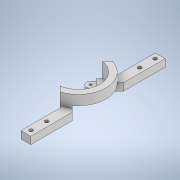
# Autodesk Inventor part: snHeadbarHolder2
Saved by Autodesk Inventor 2022 (Build 260153000, 153)
## iProperties
Created: 2022-02-24
Part Number: snHeadbarHolder2
Material: Generic
Document SubType Name: Modeling
Designer: misaa
Density: 1 g/cm^3
Appearance: Default
Author: misaa
Autodesk Inventor part; units mm, degrees
ref_plane "YZ Plane" through (0, 0, 0) normal (1, 0, 0) x (0, 1, 0)
ref_plane "XZ Plane" through (0, 0, 0) normal (0, 1, 0) x (-1, 0, 0)
ref_plane "XY Plane" through (0, 0, 0) normal (0, 0, 1) x (1, 0, 0)
sketch "Sketch1" plane through (0, 0, 0) normal (0, 1, 0) x (-1, 0, 0)
  arc A0 (-2.4004, 17.3346) -> (-2.3887, -17.3362) centre (0, 0) ccw
  arc A1 (-6.5816, 21.5159) -> (-6.5714, -21.519) centre (0, 0) ccw
  circle A2 centre (0, 10) radius 1
  circle A3 centre (0, -10) radius 1
  arc A4 (-2.3933, 7.4462) -> (2.2712, 12.663) centre (0, 10) ccw
  arc A5 (2.4002, -12.5474) -> (-2.4749, -7.5251) centre (0, -10) ccw
  line L0 (-8, 55) -> (-16, 55)
  line L1 (-16, -55) -> (-8, -55)
  line L2 (-8, -55) -> (-8, -22.9476)
  line L3 (-8, 22.9342) -> (-8, 55)
  line L4 (-16, -23.152) -> (-16, -55)
  line L5 (-8, 22.9342) -> (2.5474, 12.3868)
  line L6 (-8, 22.9342) -> (6.9163, 22.9342) construction
  line L7 (2.5474, -12.4002) -> (-8, -22.9476)
  line L8 (-2.4749, -7.5251) -> (-9.5993, -14.6496)
  circle A6 centre (-12, -50.8) radius 1.5
  circle A7 centre (-12, -38.1) radius 1.5
  circle A8 centre (-12, 50.8) radius 1.5
  circle A9 centre (-12, 38.1) radius 1.5
  line L9 (-16, 55) -> (-16, 21.0529)
  line L10 (-9.5993, -14.6496) -> (-16, -21.0503)
  line L11 (-16, -21.0503) -> (-16, -23.152)
  line L12 (-2.3933, 7.4462) -> (-16, 21.0529)
  line L13 (0, 14.9342) -> (-4.9407, 9.9935)
  line L14 (0, -14.9476) -> (-4.9487, -9.9989)
  point P0 (-9.5889, -14.6391)
  point P1 (-9.5873, 14.6401)
  dimension "d7" = 35
  dimension "d8" = 45
  dimension "d9" = 2
  dimension "d10" = 2
  dimension "d11" = 10
  dimension "d12" = 10
  dimension "d13" = 7
  dimension "d14" = 7
  dimension "d19" = 8
  dimension "d20" = 110
  dimension "d21" = 8
  dimension "d22" = 55
  dimension "d23" = 45
  dimension "d25" = 3
  dimension "d26" = 3
  dimension "d27" = 3
  dimension "d28" = 3
  dimension "d29" = 38.1
  dimension "d31" = 50.8
  constraints: 30 end point, 11 point on line, 10 centre point, 9 point on circle, 6 parallel, 4 coincident, 4 perpendicular, 2 horizontal, 1 equal length, 1 tangent, 1 vertical
  measures "d7" diameter of A0
  measures "d8" diameter of A1
  measures "d9" diameter of A2
  measures "d10" diameter of A3
  measures "d11" distance of point (0, 0) A2.centre
  measures "d12" distance of point (0, 0) A3.centre
  measures "d13" diameter of A4
  measures "d14" diameter of A5
  measures "d19" distance of L1.end L1.start
  measures "d20" distance of L1.start L0.end
  measures "d21" horizontal distance of point (0, 0) L1.end
  measures "d22" vertical distance of point (0, 0) L1.start
  measures "d23" angle of L5 L6
  measures "d25" diameter of A6
  measures "d26" diameter of A7
  measures "d27" diameter of A8
  measures "d28" diameter of A9
  measures "d29" vertical distance of point (0, 0) A7.centre
  measures "d31" vertical distance of A6.centre point (0, 0)
sketch "Sketch2" plane through (0, 0, 0) normal (0, 1, 0) x (-1, 0, 0)
  arc A0 (-2.4004, 17.3346) -> (-2.3887, -17.3362) centre (0, 0) ccw
  arc A1 (-6.5816, 21.5159) -> (-6.5714, -21.519) centre (0, 0) ccw
  circle A2 centre (0, 10) radius 1.13
  circle A3 centre (0, -10) radius 1.13
  arc A4 (-2.3933, 7.4462) -> (2.2712, 12.663) centre (0, 10) ccw
  arc A5 (2.4002, -12.5474) -> (-2.4749, -7.5251) centre (0, -10) ccw
  line L0 (-8, 55) -> (-16, 55)
  line L1 (-16, -55) -> (-8, -55)
  line L2 (-8, -55) -> (-8, -22.9476)
  line L3 (-8, 22.9342) -> (-8, 55)
  line L4 (-16, -23.152) -> (-16, -55)
  line L5 (-8, 22.9342) -> (2.5474, 12.3868)
  line L6 (-8, 22.9342) -> (6.9163, 22.9342) construction
  line L7 (2.5474, -12.4002) -> (-8, -22.9476)
  line L8 (-2.4749, -7.5251) -> (-9.5993, -14.6496)
  circle A6 centre (-12, -50.8) radius 1.5
  circle A7 centre (-12, -38.1) radius 1.5
  circle A8 centre (-12, 50.8) radius 1.5
  circle A9 centre (-12, 38.1) radius 1.5
  line L9 (-16, 55) -> (-16, 21.0529)
  line L10 (-9.5993, -14.6496) -> (-16, -21.0503)
  line L11 (-16, -21.0503) -> (-16, -23.152)
  line L12 (-2.3933, 7.4462) -> (-16, 21.0529)
  line L13 (0, 14.9342) -> (-4.9407, 9.9935)
  line L14 (0, -14.9476) -> (-4.9487, -9.9989)
  dimension "d54" = 35
  dimension "d55" = 45
  dimension "d56" = 2.26
  dimension "d57" = 2.26
  dimension "d58" = 10
  dimension "d59" = 10
  dimension "d60" = 7
  dimension "d61" = 7
  dimension "d62" = 8
  dimension "d63" = 110
  dimension "d64" = 8
  dimension "d65" = 55
  dimension "d66" = 45
  dimension "d67" = 3
  dimension "d68" = 3
  dimension "d69" = 3
  dimension "d70" = 3
  dimension "d71" = 38.1
  dimension "d72" = 50.8
  constraints: 30 end point, 11 point on line, 10 centre point, 9 point on circle, 6 parallel, 4 coincident, 4 perpendicular, 2 horizontal, 1 equal length, 1 tangent, 1 vertical
  measures "d54" diameter of A0
  measures "d55" diameter of A1
  measures "d56" diameter of A2
  measures "d57" diameter of A3
  measures "d58" distance of point (0, 0) A2.centre
  measures "d59" distance of point (0, 0) A3.centre
  measures "d60" diameter of A4
  measures "d61" diameter of A5
  measures "d62" distance of L1.end L1.start
  measures "d63" distance of L1.start L0.end
  measures "d64" horizontal distance of point (0, 0) L1.end
  measures "d65" vertical distance of point (0, 0) L1.start
  measures "d66" angle of L5 L6
  measures "d67" diameter of A6
  measures "d68" diameter of A7
  measures "d69" diameter of A8
  measures "d70" diameter of A9
  measures "d71" vertical distance of point (0, 0) A7.centre
  measures "d72" vertical distance of A6.centre point (0, 0)
sketch "Sketch3" plane through (0, 0, 0) normal (0, 1, 0) x (-1, 0, 0)
  arc A0 (-2.4004, 17.3346) -> (-2.3887, -17.3362) centre (0, 0) ccw
  arc A1 (-6.5816, 21.5159) -> (-6.5714, -21.519) centre (0, 0) ccw
  circle A2 centre (0, 10) radius 1
  circle A3 centre (0, -10) radius 1
  arc A4 (-2.3933, 7.4462) -> (2.2712, 12.663) centre (0, 10) ccw
  arc A5 (2.4002, -12.5474) -> (-2.4749, -7.5251) centre (0, -10) ccw
  line L0 (-8, 55) -> (-16, 55)
  line L1 (-16, -55) -> (-8, -55)
  line L2 (-8, -55) -> (-8, -22.9476)
  line L3 (-8, 22.9342) -> (-8, 55)
  line L4 (-16, -23.152) -> (-16, -55)
  line L5 (-8, 22.9342) -> (2.5474, 12.3868)
  line L6 (-8, 22.9342) -> (6.9163, 22.9342) construction
  line L7 (2.5474, -12.4002) -> (-8, -22.9476)
  line L8 (-2.4749, -7.5251) -> (-9.5993, -14.6496)
  circle A6 centre (-12, -50.8) radius 1.5
  circle A7 centre (-12, -38.1) radius 1.5
  circle A8 centre (-12, 50.8) radius 1.5
  circle A9 centre (-12, 38.1) radius 1.5
  line L9 (-16, 55) -> (-16, 21.0529)
  line L10 (-9.5993, -14.6496) -> (-16, -21.0503)
  line L11 (-16, -21.0503) -> (-16, -23.152)
  line L12 (-2.3933, 7.4462) -> (-16, 21.0529)
  line L13 (0, 14.9342) -> (-4.9407, 9.9935)
  line L14 (0, -14.9476) -> (-4.9487, -9.9989)
  point P0 (-9.5889, -14.6391)
  point P1 (-9.5873, 14.6401)
  point P2 (-13.1831, -18.2334)
  point P3 (-13.1816, 18.2345)
  dimension "d92" = 35
  dimension "d93" = 45
  dimension "d94" = 2
  dimension "d95" = 2
  dimension "d96" = 10
  dimension "d97" = 10
  dimension "d98" = 7
  dimension "d99" = 7
  dimension "d100" = 8
  dimension "d101" = 110
  dimension "d102" = 8
  dimension "d103" = 55
  dimension "d104" = 45
  dimension "d105" = 3
  dimension "d106" = 3
  dimension "d107" = 3
  dimension "d108" = 3
  dimension "d109" = 38.1
  dimension "d110" = 50.8
  constraints: 30 end point, 11 point on line, 10 centre point, 9 point on circle, 6 parallel, 4 coincident, 4 perpendicular, 2 horizontal, 1 equal length, 1 tangent, 1 vertical
  measures "d92" diameter of A0
  measures "d93" diameter of A1
  measures "d94" diameter of A2
  measures "d95" diameter of A3
  measures "d96" distance of point (0, 0) A2.centre
  measures "d97" distance of point (0, 0) A3.centre
  measures "d98" diameter of A4
  measures "d99" diameter of A5
  measures "d100" distance of L1.end L1.start
  measures "d101" distance of L1.start L0.end
  measures "d102" horizontal distance of point (0, 0) L1.end
  measures "d103" vertical distance of point (0, 0) L1.start
  measures "d104" angle of L5 L6
  measures "d105" diameter of A6
  measures "d106" diameter of A7
  measures "d107" diameter of A8
  measures "d108" diameter of A9
  measures "d109" vertical distance of point (0, 0) A7.centre
  measures "d110" vertical distance of A6.centre point (0, 0)
sketch "Sketch4" plane through (0, 0, 0) normal (0, 1, 0) x (-1, 0, 0)
  arc A0 (-2.4004, 17.3346) -> (-2.3887, -17.3362) centre (0, 0) ccw
  arc A1 (-6.5816, 21.5159) -> (-6.5714, -21.519) centre (0, 0) ccw
  circle A2 centre (0, 10) radius 1
  circle A3 centre (0, -10) radius 1
  arc A4 (-2.3933, 7.4462) -> (2.2712, 12.663) centre (0, 10) ccw
  arc A5 (2.4002, -12.5474) -> (-2.4749, -7.5251) centre (0, -10) ccw
  line L0 (-8, 55) -> (-16, 55)
  line L1 (-16, -55) -> (-8, -55)
  line L2 (-8, -55) -> (-8, -22.9476)
  line L3 (-8, 22.9342) -> (-8, 55)
  line L4 (-16, -23.152) -> (-16, -55)
  line L5 (-8, 22.9342) -> (2.5474, 12.3868)
  line L6 (-8, 22.9342) -> (6.9163, 22.9342) construction
  line L7 (2.5474, -12.4002) -> (-8, -22.9476)
  line L8 (-2.4749, -7.5251) -> (-9.5993, -14.6496)
  circle A6 centre (-12, -50.8) radius 1.5
  circle A7 centre (-12, -38.1) radius 1.5
  circle A8 centre (-12, 50.8) radius 1.5
  circle A9 centre (-12, 38.1) radius 1.5
  line L9 (-16, 55) -> (-16, 21.0529)
  line L10 (-9.5993, -14.6496) -> (-16, -21.0503)
  line L11 (-16, -21.0503) -> (-16, -23.152)
  line L12 (-2.3933, 7.4462) -> (-16, 21.0529)
  line L13 (0, 14.9342) -> (-4.9407, 9.9935)
  line L14 (0, -14.9476) -> (-4.9487, -9.9989)
  dimension "d35" = 35
  dimension "d36" = 45
  dimension "d37" = 2
  dimension "d38" = 2
  dimension "d39" = 10
  dimension "d40" = 10
  dimension "d41" = 7
  dimension "d42" = 7
  dimension "d43" = 8
  dimension "d44" = 110
  dimension "d45" = 8
  dimension "d46" = 55
  dimension "d47" = 45
  dimension "d48" = 3
  dimension "d49" = 3
  dimension "d50" = 3
  dimension "d51" = 3
  dimension "d52" = 38.1
  dimension "d53" = 50.8
  constraints: 30 end point, 11 point on line, 10 centre point, 9 point on circle, 6 parallel, 4 coincident, 4 perpendicular, 2 horizontal, 1 equal length, 1 tangent, 1 vertical
  measures "d35" diameter of A0
  measures "d36" diameter of A1
  measures "d37" diameter of A2
  measures "d38" diameter of A3
  measures "d39" distance of point (0, 0) A2.centre
  measures "d40" distance of point (0, 0) A3.centre
  measures "d41" diameter of A4
  measures "d42" diameter of A5
  measures "d43" distance of L1.end L1.start
  measures "d44" distance of L1.start L0.end
  measures "d45" horizontal distance of point (0, 0) L1.end
  measures "d46" vertical distance of point (0, 0) L1.start
  measures "d47" angle of L5 L6
  measures "d48" diameter of A6
  measures "d49" diameter of A7
  measures "d50" diameter of A8
  measures "d51" diameter of A9
  measures "d52" vertical distance of point (0, 0) A7.centre
  measures "d53" vertical distance of A6.centre point (0, 0)
sketch "Sketch5" plane through (0, 0, 0) normal (0, 1, 0) x (-1, 0, 0)
  arc A0 (-2.4004, 17.3346) -> (-2.3887, -17.3362) centre (0, 0) ccw
  arc A1 (-6.5816, 21.5159) -> (-6.5714, -21.519) centre (0, 0) ccw
  circle A2 centre (0, 10) radius 1
  circle A3 centre (0, -10) radius 1
  arc A4 (-2.3933, 7.4462) -> (2.2712, 12.663) centre (0, 10) ccw
  arc A5 (2.4002, -12.5474) -> (-2.4749, -7.5251) centre (0, -10) ccw
  line L0 (-8, 55) -> (-16, 55)
  line L1 (-16, -55) -> (-8, -55)
  line L2 (-8, -55) -> (-8, -22.9476)
  line L3 (-8, 22.9342) -> (-8, 55)
  line L4 (-16, -23.152) -> (-16, -55)
  line L5 (-8, 22.9342) -> (2.5474, 12.3868)
  line L6 (-8, 22.9342) -> (6.9163, 22.9342) construction
  line L7 (2.5474, -12.4002) -> (-8, -22.9476)
  line L8 (-2.4749, -7.5251) -> (-9.5993, -14.6496)
  circle A6 centre (-12, -50.8) radius 1.5
  circle A7 centre (-12, -38.1) radius 1.5
  circle A8 centre (-12, 50.8) radius 1.5
  circle A9 centre (-12, 38.1) radius 1.5
  line L9 (-16, 55) -> (-16, 21.0529)
  line L10 (-9.5993, -14.6496) -> (-16, -21.0503)
  line L11 (-16, -21.0503) -> (-16, -23.152)
  line L12 (-2.3933, 7.4462) -> (-16, 21.0529)
  line L13 (0, 14.9342) -> (-4.9407, 9.9935)
  line L14 (0, -14.9476) -> (-4.9487, -9.9989)
  point P0 (-9.5873, 14.6401)
  point P1 (-13.1816, 18.2345)
  point P2 (-13.1831, -18.2334)
  point P3 (-9.5889, -14.6391)
  dimension "d73" = 35
  dimension "d74" = 45
  dimension "d75" = 2
  dimension "d76" = 2
  dimension "d77" = 10
  dimension "d78" = 10
  dimension "d79" = 7
  dimension "d80" = 7
  dimension "d81" = 8
  dimension "d82" = 110
  dimension "d83" = 8
  dimension "d84" = 55
  dimension "d85" = 45
  dimension "d86" = 3
  dimension "d87" = 3
  dimension "d88" = 3
  dimension "d89" = 3
  dimension "d90" = 38.1
  dimension "d91" = 50.8
  constraints: 30 end point, 11 point on line, 10 centre point, 9 point on circle, 6 parallel, 4 coincident, 4 perpendicular, 2 horizontal, 1 equal length, 1 tangent, 1 vertical
  measures "d73" diameter of A0
  measures "d74" diameter of A1
  measures "d75" diameter of A2
  measures "d76" diameter of A3
  measures "d77" distance of point (0, 0) A2.centre
  measures "d78" distance of point (0, 0) A3.centre
  measures "d79" diameter of A4
  measures "d80" diameter of A5
  measures "d81" distance of L1.end L1.start
  measures "d82" distance of L1.start L0.end
  measures "d83" horizontal distance of point (0, 0) L1.end
  measures "d84" vertical distance of point (0, 0) L1.start
  measures "d85" angle of L5 L6
  measures "d86" diameter of A6
  measures "d87" diameter of A7
  measures "d88" diameter of A8
  measures "d89" diameter of A9
  measures "d90" vertical distance of point (0, 0) A7.centre
  measures "d91" vertical distance of A6.centre point (0, 0)
extrude "Extrusion1" add sketch "Sketch2" along normal blind 2 contours L5 A4 L12 L13 | L8 A5 L7 L14
extrude "Extrusion2" add sketch "Sketch1" along normal blind 4 contours L5 L13 L12 A0 | L8 L14 L7 A0
extrude "Extrusion3" add sketch "Sketch3" along normal blind 6 contours A1 L12 L9 L0 L3 L5 | A1 L7 L2 L1 L4 L11 L10
extrude "Extrusion4" add sketch "Sketch4" along normal blind 16 contours A0 L12 A1 L5 | A0 L8 L10 A1 L12 | A0 L7 A1 L10 L8
extrude "Extrusion5" cut sketch "Sketch5" along normal blind 8 contours A0 L8 L10 A1 L12
thread "Thread1" size "4-40 UNC" class "2B" standard "ANSI Unified Screw Threads" full length
thread "Thread2" size "4-40 UNC" class "2B" standard "ANSI Unified Screw Threads" full length
body "Solid1"
